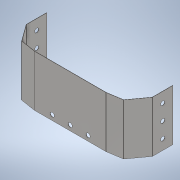
# Autodesk Inventor part: New front
Saved by Autodesk Inventor 2020 (Build 240168000, 168)
## iProperties
Created: 2022-07-17
Part Number: New front
Material: Generic
Document SubType Name: Sheet Metal
Designer: karimi2
Density: 1 g/cm^3
Sheet Metal Rule: Default_mm
Appearance: Steel - Polished
Author: karimi2
Autodesk Inventor part; units mm, degrees
ref_plane "YZ Plane" through (0, 0, 0) normal (1, 0, 0) x (0, 1, 0)
ref_plane "XZ Plane" through (0, 0, 0) normal (0, 1, 0) x (-1, 0, 0)
ref_plane "XY Plane" through (0, 0, 0) normal (0, 0, 1) x (1, 0, 0)
sketch "Sketch1" plane through (0, 0, 0) normal (0, 0, 1) x (1, 0, 0)
  line L0 (-140, 0) -> (-140, 100)
  line L1 (-140, 100) -> (0, 100)
  line L2 (0, 100) -> (0, 0) construction
  line L3 (-140, 0) -> (-70, 0)
  line L4 (-100, 100) -> (-100, 0)
  line L5 (-70, 100) -> (-70, 0)
  line L6 (140, 0) -> (140, 100)
  line L7 (140, 100) -> (0, 100)
  line L8 (140, 0) -> (70, 0)
  line L9 (100, 100) -> (100, 0)
  line L10 (70, 100) -> (70, 0)
  line L11 (-70, 0) -> (70, 0)
  line L12 (140, 100) -> (180, 100)
  line L13 (180, 100) -> (180, 0)
  line L14 (180, 0) -> (140, 0)
  line L15 (-140, 100) -> (-180, 100)
  line L16 (-180, 100) -> (-180, 0)
  line L17 (-180, 0) -> (-140, 0)
  dimension "d121" = 100
  dimension "d122" = 360
  dimension "d123" = 40
  dimension "d124" = 80
  dimension "d125" = 110
  dimension "d126" = 180
  dimension "d127" = 100
  dimension "d128" = 110
  constraints: 36 end point, 8 point on line, 7 symmetric about line, 5 perpendicular, 3 horizontal, 2 midpoint, 2 parallel, 1 vertical
  measures "d121" distance from line of L2.end L7
  measures "d122" distance between parallel lines of L13 L16
  measures "d123" distance between parallel lines of L6 L13
  measures "d124" distance between parallel lines of L9 L13
  measures "d125" distance between parallel lines of L10 L13
  measures "d126" distance between parallel lines of L13 L2
  measures "d127" distance between parallel lines of L17 L15
  measures "d128" distance from line of L8.end L13
extrude "Plate3" add sketch "Sketch1" along normal blind 0.5
fold "Fold13" angle 36 bend radius 0.5 thickness 0.5 k factor 0.44 line from (-140, 0, 0) to (-140, 100, 0) line at bend centre moving side (-1, 0, 0) folds toward (0, 0, -1)
fold "Fold14" angle 45 bend radius 0.5 thickness 0.5 k factor 0.44 line from (-100, 100, 0) to (-100, 0, 0) line at bend centre moving side (-1, 0, 0) folds toward (0, 0, -1)
fold "Fold15" angle 36 bend radius 0.5 thickness 0.5 k factor 0.44 line from (140, 0, 0) to (140, 100, 0) line at bend centre moving side (1, 0, 0) folds toward (0, 0, -1)
fold "Fold16" angle 45 bend radius 0.5 thickness 0.5 k factor 0.44 line from (100, 100, 0) to (100, 0, 0) line at bend centre moving side (1, 0, 0) folds toward (0, 0, -1)
fold "Fold17" angle 9 bend radius 0.5 thickness 0.5 k factor 0.44 line from (-70, 100, 0) to (-70, 0, 0) line at bend centre moving side (-1, 0, 0) folds toward (0, 0, -1)
fold "Fold18" angle 9 bend radius 0.5 thickness 0.5 k factor 0.44 line from (70, 100, 0) to (70, 0, 0) line at bend centre moving side (1, 0, 0) folds toward (0, 0, -1)
sketch "Sketch8" plane through (123.4513, 0, -76.8627) normal (1, 0, 0) x (0, 0, -1)
  line L0 (-39.7738, 100) -> (0, 100) projected
  line L1 (0, 100) -> (0, 0) projected
  point P0 (-76.8627, 0)
  point P1 (-20, 80)
  point P2 (-20, 50)
  point P3 (-20, 20)
  dimension "d173" = 20
  dimension "d174" = 50
  dimension "d175" = 80
  dimension "d176" = 20
  constraints: 2 vertical alignment
  measures "d173" distance from line of L0 point (-20, 80)
  measures "d174" distance from line of point (-20, 50) L0
  measures "d175" distance from line of point (-20, 20) L0
  measures "d176" distance from line of L1 point (-20, 80)
hole "Hole4" at (123.4513, 80, -56.8627) at (123.4513, 50, -56.8627) at (123.4513, 20, -56.8627) direction (-1, 0, 0) diameter 8 end through all
sketch "Sketch9" plane through (0, 0, 0.5) normal (0, 0, 1) x (1, 0, 0)
  line L0 (-69.9435, 100) -> (-69.9435, 0) projected
  line L1 (69.9435, 0) -> (-69.9435, 0) projected
  point P0 (0, 0)
  point P1 (-34.9435, 10)
  point P2 (0.0565, 10)
  point P3 (35.0565, 10)
  dimension "d184" = 35
  dimension "d185" = 35
  dimension "d186" = 35
  dimension "d187" = 10
  constraints: 2 horizontal alignment
  measures "d184" distance from line of L0 point (-34.943, 10)
  measures "d185" distance of point (0.057, 10) point (-34.943, 10)
  measures "d186" distance of point (35.057, 10) point (0.057, 10)
  measures "d187" distance from line of L1 point (-34.943, 10)
hole "Hole5" at (-34.9435, 10, 0.5) at (0.0565, 10, 0.5) at (35.0565, 10, 0.5) direction (0, 0, -1) diameter 8 end through all
equation "\"d129\" = Thickness"
equation "\"d130\" = BendReliefWidth"
equation "\"d131\" = BendReliefDepth"
equation "\"d132\" = MinimumRemnant"
equation "\"d133\" = TransitionRadius"
equation "\"d135\" = BendRadius"
equation "\"d136\" = BendReliefWidth"
equation "\"d137\" = BendReliefDepth"
equation "\"d138\" = MinimumRemnant"
equation "\"d139\" = TransitionRadius"
equation "\"d141\" = BendRadius"
equation "\"d142\" = BendReliefWidth"
equation "\"d143\" = BendReliefDepth"
equation "\"d144\" = MinimumRemnant"
equation "\"d145\" = TransitionRadius"
equation "\"d147\" = BendRadius"
equation "\"d148\" = BendReliefWidth"
equation "\"d149\" = BendReliefDepth"
equation "\"d150\" = MinimumRemnant"
equation "\"d151\" = TransitionRadius"
equation "\"d153\" = BendRadius"
equation "\"d154\" = BendReliefWidth"
equation "\"d155\" = BendReliefDepth"
equation "\"d156\" = MinimumRemnant"
equation "\"d157\" = TransitionRadius"
equation "\"d159\" = BendRadius"
equation "\"d160\" = BendReliefWidth"
equation "\"d161\" = BendReliefDepth"
equation "\"d162\" = MinimumRemnant"
equation "\"d163\" = TransitionRadius"
equation "\"d165\" = BendRadius"
equation "\"d171\" = Thickness"
equation "\"d182\" = Thickness"
equation "\"BendRadius\" = Thickness"
equation "\"BendReliefWidth\" = Thickness"
equation "\"BendReliefDepth\" = 0.5 * Thickness"
equation "\"CornerReliefSize\" = 4 * Thickness"
equation "\"MinimumRemnant\" = 2 * Thickness"
equation "\"TransitionRadius\" = BendRadius"
equation "\"JacobiRadiusSize\" = BendRadius"
equation "\"GapSize\" = Thickness"
equation "\"Thickness\" = 0.5"
body "Solid3"
